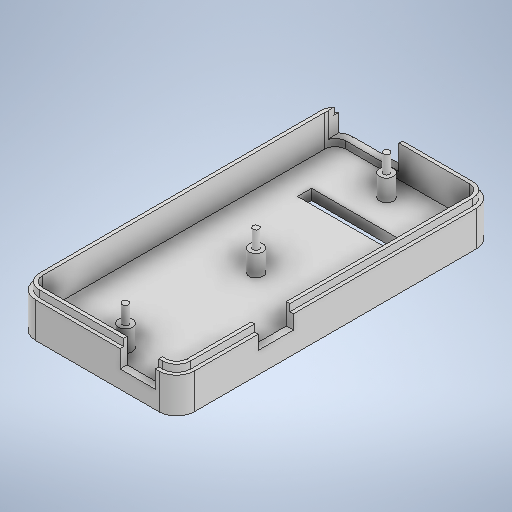
# Autodesk Inventor part: Pieza_superior
Saved by Autodesk Inventor 2025.1 (Build 291241000, 241)
## iProperties
Created: 2024-08-25
Part Number: Pieza_superior
Material: Genérico
Document SubType Name: Modeling
Designer: User
Density: 1 g/cm^3
Appearance: Valor por defecto
Author: User
Autodesk Inventor part; units mm, degrees
ref_plane "YZ Plane" through (0, 0, 0) normal (1, 0, 0) x (0, 1, 0)
ref_plane "XZ Plane" through (0, 0, 0) normal (0, 1, 0) x (-1, 0, 0)
ref_plane "XY Plane" through (0, 0, 0) normal (0, 0, 1) x (1, 0, 0)
sketch "Boceto1" plane through (0, 0, 0) normal (0, 1, 0) x (-1, 0, 0)
  line L0 (17.5, 45) -> (-17.5, 45)
  line L1 (-22.5, 40) -> (-22.5, -40)
  line L2 (-17.5, -45) -> (17.5, -45)
  line L3 (22.5, -40) -> (22.5, 40)
  line L4 (22.5, 45) -> (-22.5, -45) construction
  line L5 (-22.5, 45) -> (22.5, -45) construction
  arc A0 (22.5, 40) -> (17.5, 45) centre (17.5, 40) ccw
  arc A1 (-17.5, 45) -> (-22.5, 40) centre (-17.5, 40) ccw
  arc A2 (-22.5, -40) -> (-17.5, -45) centre (-17.5, -40) ccw
  arc A3 (17.5, -45) -> (22.5, -40) centre (17.5, -40) ccw
  point P0 (0, 0)
  dimension "d0" = 45
  dimension "d1" = 90
  dimension "d2" = 5
  constraints: 12 end point, 8 point on circle, 8 point on line, 8 tangent, 4 centre point, 3 equal radius, 2 midpoint, 2 parallel, 1 horizontal, 1 perpendicular
  measures "d0" distance of L5.end L4.end
  measures "d1" distance of L4.end L5.start
  measures "d2" radius of A0
extrude "Extrusión1" add sketch "Boceto1" along normal blind 10
sketch "Boceto3" plane through (0, 10, 0) normal (0, 1, 0) x (1, 0, 0)
  line L0 (17.5, 43) -> (-17.5, 43) projected
  arc A0 (-17.5, 43) -> (-20.5, 40) centre (-17.5, 40) ccw projected
  line L1 (-20.5, 40) -> (-20.5, -40) projected
  arc A1 (-20.5, -40) -> (-17.5, -43) centre (-17.5, -40) ccw projected
  line L2 (-17.5, -43) -> (17.5, -43) projected
  arc A2 (17.5, -43) -> (20.5, -40) centre (17.5, -40) ccw projected
  line L3 (20.5, -40) -> (20.5, 40) projected
  arc A3 (20.5, 40) -> (17.5, 43) centre (17.5, 40) ccw projected
  point P0 (0, 0)
extrude "Extrusión3" cut sketch "Boceto3" against normal blind 7
sketch "Boceto5" plane through (0, 3, 0) normal (0, 1, 0) x (1, 0, 0)
  circle A0 centre (0, 0) radius 2
  dimension "d21" = 4
  constraints: 1 centre point, 1 coincident
  measures "d21" diameter of A0
extrude "Extrusión5" add sketch "Boceto5" along normal blind 6
sketch "Boceto6" plane through (0, 9, 0) normal (0, 1, 0) x (1, 0, 0)
  circle A0 centre (0, 0) radius 2 projected
  circle A1 centre (0, 0) radius 0.9
  dimension "d24" = 1.8
  constraints: 1 centre point, 1 coincident
  measures "d24" diameter of A1
extrude "Extrusión6" add sketch "Boceto6" along normal blind 5 contours A1
sketch "Boceto7" plane through (0, 10, 0) normal (0, 1, 0) x (1, 0, 0)
  line L0 (-20.5, -40) -> (-20.5, 40) projected
  arc A0 (-17.5, 43) -> (-20.5, 40) centre (-17.5, 40) ccw projected
  line L1 (-17.5, 43) -> (17.5, 43) projected
  arc A1 (20.5, 40) -> (17.5, 43) centre (17.5, 40) ccw projected
  line L2 (20.5, 40) -> (20.5, -40) projected
  arc A2 (17.5, -43) -> (20.5, -40) centre (17.5, -40) ccw projected
  line L3 (17.5, -43) -> (-17.5, -43) projected
  arc A3 (-20.5, -40) -> (-17.5, -43) centre (-17.5, -40) ccw projected
  arc A4 (17.5, -45) -> (22.5, -40) centre (17.5, -40) ccw projected
  line L4 (22.5, -40) -> (22.5, 40) projected
  arc A5 (22.5, 40) -> (17.5, 45) centre (17.5, 40) ccw projected
  line L5 (17.5, 45) -> (-17.5, 45) projected
  arc A6 (-17.5, 45) -> (-22.5, 40) centre (-17.5, 40) ccw projected
  line L6 (-22.5, 40) -> (-22.5, -40) projected
  arc A7 (-22.5, -40) -> (-17.5, -45) centre (-17.5, -40) ccw projected
  line L7 (-17.5, -45) -> (17.5, -45) projected
  line L8 (-17.5, -44) -> (17.5, -44)
  arc A8 (17.5, -44) -> (21.5, -40) centre (17.5, -40) ccw
  line L9 (21.5, -40) -> (21.5, 40)
  arc A9 (21.5, 40) -> (17.5, 44) centre (17.5, 40) ccw
  line L10 (17.5, 44) -> (-17.5, 44)
  arc A10 (-17.5, 44) -> (-21.5, 40) centre (-17.5, 40) ccw
  line L11 (-21.5, 40) -> (-21.5, -40)
  arc A11 (-21.5, -40) -> (-17.5, -44) centre (-17.5, -40) ccw
  point P0 (0, 0)
  dimension "d27" = 1
  constraints: 8 end point, 8 point on circle, 4 centre point, 7 other
  measures "d27" radial gap between concentric circles of A3 A11
extrude "Extrusión7" add sketch "Boceto7" along normal blind 2 contours A11 L11 A10 L10 A9 L9 A8 L8
sketch "Boceto8" plane through (0, 3, 0) normal (0, 1, 0) x (1, 0, 0)
  line L0 (17.5, -43) -> (-17.5, -43) construction
  line L1 (0, -43) -> (0, -37) construction
  line L2 (-17.5, 43) -> (17.5, 43) construction
  line L3 (0, 43) -> (0, 37) construction
  circle A0 centre (0, -37) radius 2
  circle A1 centre (0, -37) radius 1.5
  circle A2 centre (0, 37) radius 2
  circle A3 centre (0, 37) radius 1.5
  point P0 (0, 0)
  dimension "d30" = 6
  dimension "d31" = 6
  dimension "d32" = 4
  dimension "d33" = 3
  dimension "d34" = 4
  dimension "d35" = 3
  constraints: 4 centre point, 4 coincident, 4 end point, 2 midpoint, 2 vertical
  measures "d30" distance of L1.start L1.end
  measures "d31" distance of L3.start L3.end
  measures "d32" diameter of A0
  measures "d33" diameter of A1
  measures "d34" diameter of A2
  measures "d35" diameter of A3
extrude "Extrusión8" add sketch "Boceto8" along normal blind 6 contours A0 | A1 | A2 | A3
sketch "Boceto9" plane through (0, 0, 0) normal (0, -1, 0) x (1, 0, 0)
  line L0 (0, -28.5) -> (23, -28.5) construction
  line L1 (0, -28.5) -> (0, -24.5) construction
  line L2 (12.75, -24.5) -> (-12.75, -24.5)
  line L3 (-12.75, -24.5) -> (-12.75, -28.5)
  line L4 (-12.75, -28.5) -> (12.75, -28.5)
  line L5 (12.75, -28.5) -> (12.75, -24.5)
  line L6 (12.75, -24.5) -> (-12.75, -28.5) construction
  line L7 (-12.75, -24.5) -> (12.75, -28.5) construction
  point P0 (0, 0)
  point P1 (0, -26.5)
  dimension "d38" = 4
  dimension "d39" = 25.5
  constraints: 16 end point, 3 midpoint, 2 horizontal, 2 parallel, 1 perpendicular, 1 vertical
  measures "d38" distance of L0.start L1.end
  measures "d39" distance of L4.end L3.end
extrude "Extrusión9" cut sketch "Boceto9" against normal blind 10
sketch "Sketch10" plane through (0, 9, -37) normal (0, 1, 0) x (1, 0, 0)
  circle A0 centre (0, 0) radius 0.9
  point P0 (0, -37)
  dimension "d42" = 1.8
  constraints: 1 centre point
  measures "d42" diameter of A0
extrude "Extrusion10" add sketch "Sketch10" along normal blind 5
sketch "Sketch11" plane through (0, 9, 37) normal (0, 1, 0) x (1, 0, 0)
  circle A0 centre (0, 0) radius 0.9
  point P0 (0, 37)
  dimension "d45" = 1.8
  constraints: 1 centre point
  measures "d45" diameter of A0
extrude "Extrusion11" add sketch "Sketch11" along normal blind 5
sketch "Sketch15" plane through (17.5, 0, -45) normal (0, 0, -1) x (-1, 0, 0)
  line L0 (38.0046, 12.0013) -> (20.0046, 12.0013)
  line L1 (20.0046, 12.0013) -> (20.0046, 5.0013)
  line L2 (20.0046, 5.0013) -> (38.0046, 5.0013)
  line L3 (38.0046, 5.0013) -> (38.0046, 12.0013)
  point P0 (17.5, 0)
  dimension "d50" = 18
  dimension "d51" = 7
  constraints: 8 end point, 2 parallel, 1 horizontal, 1 perpendicular
  measures "d50" distance of L2.end L1.end
  measures "d51" distance of L1.end L0.end
extrude "Extrusion12" cut sketch "Sketch15" against normal blind 4
sketch "Sketch17" plane through (22.5, 0, 40) normal (1, 0, 0) x (0, 0, -1)
  line L0 (0, 12) -> (80, 12) projected
  line L1 (18.1121, 12) -> (28.1121, 12)
  line L2 (28.1121, 12) -> (28.1121, 6)
  line L3 (28.1121, 6) -> (18.1121, 6)
  line L4 (18.1121, 6) -> (18.1121, 12)
  point P0 (40, 0)
  dimension "d56" = 10
  dimension "d57" = 6
  constraints: 8 end point, 2 parallel, 1 horizontal, 1 perpendicular, 1 point on line
  measures "d56" distance of L2.end L3.end
  measures "d57" distance of L1.end L2.end
extrude "Extrusion13" cut sketch "Sketch17" against normal blind 4
sketch "Sketch18" plane through (-17.5, 0, 45) normal (0, 0, 1) x (1, 0, 0)
  line L0 (33.9645, 12) -> (23.9645, 12)
  line L1 (23.9645, 12) -> (23.9645, 5)
  line L2 (23.9645, 5) -> (33.9645, 5)
  line L3 (33.9645, 5) -> (33.9645, 12)
  point P0 (17.5, 0)
  dimension "d60" = 10
  dimension "d61" = 7
  constraints: 8 end point, 2 parallel, 1 horizontal, 1 perpendicular
  measures "d60" distance of L2.end L1.end
  measures "d61" distance of L1.end L0.end
extrude "Extrusion14" cut sketch "Sketch18" against normal blind 4
